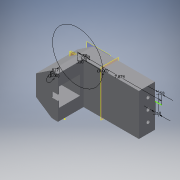
# Autodesk Inventor part: ZFrame
Saved by Autodesk Inventor 2016 (Build 200138000, 138)
## iProperties
Created: 2016-03-26
Part Number: ZFrame
Material: Generic
Document SubType Name: Modeling
Designer: Scott
Density: 1 g/cm^3
Appearance: Default
Author: Scott
Autodesk Inventor part; units mm, degrees
ref_plane "YZ Plane" through (0, 0, 0) normal (1, 0, 0) x (0, 1, 0)
ref_plane "XZ Plane" through (0, 0, 0) normal (0, 1, 0) x (-1, 0, 0)
ref_plane "XY Plane" through (0, 0, 0) normal (0, 0, 1) x (1, 0, 0)
ref_plane "Work Plane1" through (-25.4, 50.8, 0) normal (0, 1, 0) x (0, 0, -1)
ref_plane "Work Plane2" through (0, 0, 0) normal (0, 0, 1) x (1, 0, 0)
sketch "Sketch1" plane through (0, 0, 0) normal (0, 0, 1) x (1, 0, 0)
  point P0 (0, 0)
ref_plane "Work Plane3" through (0, 0, 3.175) normal (0, 0, 1) x (1, 0, 0)
sketch "Sketch2" plane through (0, 0, 3.175) normal (0, 0, 1) x (1, 0, 0)
  arc A0 (-27.2599, 1.8599) -> (-22.7697, 0) centre (-22.7697, 6.35) ccw projected
  line L0 (-27.2599, 1.8599) -> (-48.9401, 23.5401) projected
  arc A1 (-50.8, 28.0303) -> (-48.9401, 23.5401) centre (-44.45, 28.0303) ccw projected
  line L1 (-50.8, 28.0303) -> (-50.8, 48.1697) projected
  arc A2 (-48.9401, 52.6599) -> (-50.8, 48.1697) centre (-44.45, 48.1697) ccw projected
  line L2 (-48.9401, 52.6599) -> (-27.2599, 74.3401) projected
  arc A3 (-22.7697, 76.2) -> (-27.2599, 74.3401) centre (-22.7697, 69.85) ccw projected
  line L3 (-22.7697, 76.2) -> (0, 76.2) projected
  line L4 (0, 76.2) -> (0, 0) projected
  line L5 (0, 0) -> (-22.7697, 0) projected
  arc A4 (-25.4, 0.5704) -> (-22.7697, 0) centre (-22.7697, 6.35) ccw projected
  line L6 (0, 0) -> (-22.7697, 0) projected
  line L7 (0, 76.2) -> (0, 0) projected
  line L8 (0, 76.2) -> (-22.7697, 76.2) projected
  arc A5 (-22.7697, 76.2) -> (-25.4, 75.6296) centre (-22.7697, 69.85) ccw projected
  line L9 (-25.4, 57.15) -> (-25.4, 75.6296) projected
  arc A6 (-31.75, 50.8) -> (-25.4, 57.15) centre (-31.75, 57.15) ccw projected
  line L10 (-31.75, 50.8) -> (-50.2296, 50.8) projected
  arc A7 (-50.2296, 50.8) -> (-50.8, 48.1697) centre (-44.45, 48.1697) ccw projected
  line L11 (-50.8, 28.0303) -> (-50.8, 48.1697) projected
  arc A8 (-50.8, 28.0303) -> (-50.2296, 25.4) centre (-44.45, 28.0303) ccw projected
  line L12 (-31.75, 25.4) -> (-50.2296, 25.4) projected
  arc A9 (-25.4, 19.05) -> (-31.75, 25.4) centre (-31.75, 19.05) ccw projected
  line L13 (-25.4, 0.5704) -> (-25.4, 19.05) projected
  arc A10 (-22.7697, 78.74) -> (-27.94, 77.0819) centre (-22.7697, 69.85) ccw
  line L14 (-27.94, 77.0819) -> (-27.94, 57.15)
  arc A11 (-31.75, 53.34) -> (-27.94, 57.15) centre (-31.75, 57.15) ccw
  line L15 (-31.75, 53.34) -> (-51.6819, 53.34)
  line L16 (-51.6819, 22.86) -> (-31.75, 22.86)
  arc A12 (-27.94, 19.05) -> (-31.75, 22.86) centre (-31.75, 19.05) ccw
  line L17 (-27.94, 19.05) -> (-27.94, -0.8819)
  arc A13 (-27.94, -0.8819) -> (-22.7697, -2.54) centre (-22.7697, 6.35) ccw
  line L18 (-51.6819, 22.86) -> (-55.3326, 22.86)
  line L19 (-57.15, 38.1) -> (-57.15, 22.86)
  line L20 (-57.15, 22.86) -> (-55.3326, 22.86)
  line L21 (-57.15, 38.1) -> (-57.15, 53.34)
  line L22 (-57.15, 53.34) -> (-51.6819, 53.34)
  line L23 (-22.7697, -2.54) -> (0, -2.54)
  line L24 (0, -2.54) -> (117.094, -2.54)
  line L25 (-22.7697, 78.74) -> (0, 78.74)
  line L26 (0, 78.74) -> (117.094, 78.74)
  line L27 (117.094, 78.74) -> (117.094, -2.54)
  line L28 (-66.04, 62.23) -> (-66.04, 38.1)
  line L29 (-66.04, 38.1) -> (-66.04, 13.97)
  arc A14 (-36.83, -4.5329) -> (-22.7697, -11.43) centre (-22.7697, 6.35) ccw
  line L30 (-22.7697, -11.43) -> (0, -11.43)
  line L31 (0, -11.43) -> (125.984, -11.43)
  line L32 (125.984, -11.43) -> (125.984, 87.63)
  line L33 (125.984, 87.63) -> (0, 87.63)
  line L34 (0, 87.63) -> (-22.7697, 87.63)
  line L35 (-66.04, 13.97) -> (-30.6001, -9.6129)
  line L36 (-66.04, 62.23) -> (-32.6758, 84.6148)
  arc A15 (-22.7697, 87.63) -> (-32.6758, 84.6148) centre (-22.7697, 69.85) ccw
  line L37 (-48.26, 22.86) -> (-31.75, 22.86)
  line L38 (-31.75, 22.86) -> (-27.94, 19.05)
  line L39 (-27.94, 19.05) -> (-27.94, -0.8819)
  line L40 (-27.94, -0.8819) -> (-22.7697, -2.54)
  line L41 (-22.7697, 78.74) -> (-27.94, 77.0819)
  line L42 (-27.94, 77.0819) -> (-27.94, 57.15)
  line L43 (-27.94, 57.15) -> (-31.75, 53.34)
  line L44 (-31.75, 53.34) -> (-51.6819, 53.34)
  dimension "d0" = 2.54
  dimension "d1" = 2.54
  dimension "d10" = 117.094
  dimension "d11" = 180
  dimension "d12" = 117.094
  dimension "d13" = 8.89
  constraints: 62 end point, 14 point on circle, 6 centre point, 5 collinear, 4 perpendicular, 4 point on line, 2 horizontal, 2 parallel, 2 tangent, 12 other
  measures "d0" radial gap between concentric circles of A6 A11
  measures "d1" distance between parallel lines of L12 L16
  measures "d10" distance of L23.end L24.end
  measures "d11" angle of L24 L23
  measures "d12" distance of L25.end L26.end
  measures "d13" distance between parallel lines of L21 L28
ref_plane "Work Plane4" through (-20.32, 38.1, -38.1) normal (0, 0, -1) x (-1, 0, 0)
sketch "Sketch3" plane through (-20.32, 38.1, -38.1) normal (0, 0, -1) x (-1, 0, 0)
  line L0 (33.1588, 0) -> (36.9688, 0)
  line L1 (36.9688, 0) -> (45.8588, 0)
  line L2 (45.8588, 0) -> (54.7488, 0)
  line L3 (54.7488, 0) -> (-145.2512, 0)
  line L4 (-145.2512, 0) -> (-138.9012, 0)
  line L5 (-138.9012, 0) -> (-130.0112, 0)
  point P0 (-20.32, -38.1)
  dimension "d2" = 3.81
  dimension "d3" = 8.89
  dimension "d4" = 8.89
  dimension "d5" = 200
  dimension "d6" = 0
  dimension "d8" = 6.35
  dimension "d9" = 8.89
  constraints: 12 end point, 3 point on line, 2 horizontal, 1 collinear
  measures "d2" distance of L0.start L0.end
  measures "d3" distance of L0.end L1.end
  measures "d4" distance of L1.end L2.end
  measures "d5" distance of L2.end L3.end
  measures "d6" distance between parallel lines of L3 L2
  measures "d8" distance of L3.end L4.end
  measures "d9" distance of L4.end L5.end
extrude "Extrusion1" add sketch "Sketch2" against normal blind 31.75 contours L0 L17 A12 L16 A1 L12 A9 L13 A0 | L0 L16 L38 L17 | L38 A12 | L9 A6 L10 A2 L2 L15 A11 L14 A3 | L14 L43 L15 L2 | A11 L43 | L36 A15 L34 L33 L32 L31 L30 A14 L35 L29 L28
sketch "Sketch4" plane through (0, 0, -28.575) normal (0, 0, -1) x (-1, 0, 0)
  line L0 (31.75, 22.86) -> (27.94, 19.05) projected
  arc A0 (31.75, 22.86) -> (27.94, 19.05) centre (31.75, 19.05) ccw projected
  line L1 (66.04, 13.97) -> (66.04, 62.23) projected
  line L2 (66.04, 62.23) -> (32.6758, 84.6148) projected
  arc A1 (32.6758, 84.6148) -> (22.7697, 87.63) centre (22.7697, 69.85) ccw projected
  line L3 (22.7697, 87.63) -> (-125.984, 87.63) projected
  line L4 (-125.984, 87.63) -> (-125.984, -11.43) projected
  line L5 (-125.984, -11.43) -> (22.7697, -11.43) projected
  arc A2 (22.7697, -11.43) -> (30.6001, -9.6129) centre (22.7697, 6.35) ccw projected
  line L6 (30.6001, -9.6129) -> (66.04, 13.97) projected
  line L7 (27.2599, 74.3401) -> (27.94, 73.66) projected
  arc A3 (27.2599, 74.3401) -> (25.4, 75.6296) centre (22.7697, 69.85) ccw projected
  line L8 (25.4, 57.15) -> (25.4, 75.6296) projected
  arc A4 (25.4, 57.15) -> (31.75, 50.8) centre (31.75, 57.15) ccw projected
  line L9 (50.2296, 50.8) -> (31.75, 50.8) projected
  arc A5 (50.2296, 50.8) -> (48.9401, 52.6599) centre (44.45, 48.1697) ccw projected
  line L10 (48.26, 53.34) -> (48.9401, 52.6599) projected
  line L11 (48.26, 53.34) -> (57.15, 53.34) projected
  line L12 (57.15, 53.34) -> (57.15, 22.86) projected
  line L13 (57.15, 22.86) -> (48.26, 22.86) projected
  line L14 (48.9401, 23.5401) -> (48.26, 22.86) projected
  arc A6 (48.9401, 23.5401) -> (50.2296, 25.4) centre (44.45, 28.0303) ccw projected
  line L15 (31.75, 25.4) -> (50.2296, 25.4) projected
  arc A7 (31.75, 25.4) -> (25.4, 19.05) centre (31.75, 19.05) ccw projected
  line L16 (25.4, 0.5704) -> (25.4, 19.05) projected
  arc A8 (25.4, 0.5704) -> (27.2599, 1.8599) centre (22.7697, 6.35) ccw projected
  line L17 (27.94, 2.54) -> (27.2599, 1.8599) projected
  line L18 (27.94, 2.54) -> (27.94, -0.8819) projected
  arc A9 (22.7697, -2.54) -> (27.94, -0.8819) centre (22.7697, 6.35) ccw projected
  line L19 (22.7697, -2.54) -> (-117.094, -2.54) projected
  line L20 (-117.094, -2.54) -> (-117.094, 78.74) projected
  line L21 (-117.094, 78.74) -> (22.7697, 78.74) projected
  arc A10 (27.94, 77.0819) -> (22.7697, 78.74) centre (22.7697, 69.85) ccw projected
  line L22 (27.94, 77.0819) -> (27.94, 73.66) projected
  line L23 (27.94, 57.15) -> (31.75, 53.34) projected
  arc A11 (27.94, 57.15) -> (31.75, 53.34) centre (31.75, 57.15) ccw projected
  line L24 (27.94, 19.05) -> (27.94, 2.54)
  line L25 (31.75, 22.86) -> (48.26, 22.86)
  line L26 (48.26, 53.34) -> (31.75, 53.34)
  line L27 (27.94, 73.66) -> (27.94, 77.0819) projected
  line L28 (27.94, 57.15) -> (27.94, 73.66)
  point P0 (0, 0)
  constraints: 8 end point, 1 collinear, 1 horizontal, 1 perpendicular, 1 vertical
extrude "Extrusion2" cut sketch "Sketch4" against normal blind 31.75 contours A0 L24 L17 A8 L16 A7 L15 A6 L14 L25 | L10 A5 L9 A4 L8 A3 L7 L28 A11 L26
sketch "Sketch5" plane through (0, 0, -28.575) normal (0, 0, -1) x (-1, 0, 0)
  line L0 (66.04, 13.97) -> (66.04, 62.23) projected
  line L1 (66.04, 62.23) -> (32.6758, 84.6148) projected
  arc A0 (32.6758, 84.6148) -> (22.7697, 87.63) centre (22.7697, 69.85) ccw projected
  line L2 (22.7697, 87.63) -> (-125.984, 87.63) projected
  line L3 (-125.984, 87.63) -> (-125.984, -11.43) projected
  line L4 (-125.984, -11.43) -> (22.7697, -11.43) projected
  arc A1 (22.7697, -11.43) -> (30.6001, -9.6129) centre (22.7697, 6.35) ccw projected
  line L5 (30.6001, -9.6129) -> (66.04, 13.97) projected
  line L6 (57.15, 22.86) -> (31.75, 22.86) projected
  line L7 (31.75, 22.86) -> (27.94, 19.05) projected
  line L8 (27.94, 19.05) -> (27.94, -0.8819) projected
  arc A2 (22.7697, -2.54) -> (27.94, -0.8819) centre (22.7697, 6.35) ccw projected
  line L9 (22.7697, -2.54) -> (-117.094, -2.54) projected
  line L10 (-117.094, -2.54) -> (-117.094, 78.74) projected
  line L11 (-117.094, 78.74) -> (22.7697, 78.74) projected
  arc A3 (27.94, 77.0819) -> (22.7697, 78.74) centre (22.7697, 69.85) ccw projected
  line L12 (27.94, 77.0819) -> (27.94, 57.15) projected
  line L13 (27.94, 57.15) -> (31.75, 53.34) projected
  line L14 (31.75, 53.34) -> (57.15, 53.34) projected
  line L15 (57.15, 53.34) -> (57.15, 22.86) projected
  arc A4 (27.94, 57.15) -> (31.75, 53.34) centre (31.75, 57.15) ccw
  line L16 (31.75, 22.86) -> (27.94, 19.05) projected
  arc A5 (31.75, 22.86) -> (27.94, 19.05) centre (31.75, 19.05) ccw
  point P0 (0, 0)
  dimension "d18" = 3.81
  constraints: 4 point on circle, 2 centre point, 2 tangent
  measures "d18" radius of A5
extrude "Extrusion3" add sketch "Sketch5" against normal blind 31.75 contours L7 A5 | A4 L13
fillet "Fillet1" radius 3.7084 6 edges at (-29.0559, 21.7441, -28.575) (-27.94, 9.084, -28.575) (-44.45, 22.86, -28.575) (-29.0559, 54.4559, -28.575) (-27.94, 67.116, -28.575) (-40.005, 53.34, -28.575)
sketch "Sketch6" plane through (-27.94, 57.15, 3.175) normal (1, 0, 0) x (0, 0, -1)
  circle A0 centre (15.875, -44.45) radius 8 projected
  circle A1 centre (15.875, 6.35) radius 8 projected
  circle A2 centre (15.875, -44.45) radius 4
  circle A3 centre (15.875, 6.35) radius 4
  point P0 (3.175, -57.15)
  dimension "d22" = 8
  dimension "d23" = 8
  constraints: 2 centre point, 2 coincident
  measures "d22" diameter of A2
  measures "d23" diameter of A3
extrude "Extrusion4" cut sketch "Sketch6" along normal mid plane 4318 contours A2 | A3
sketch "Sketch7" plane through (117.094, -2.54, 3.175) normal (-1, 0, 0) x (0, 0, 1)
  circle A0 centre (-15.875, 40.64) radius 5.08 projected
  circle A1 centre (-15.875, 40.64) radius 4
  point P0 (-3.175, 2.54)
  dimension "d26" = 8
  constraints: 1 centre point, 1 coincident
  measures "d26" diameter of A1
extrude "Extrusion5" cut sketch "Sketch7" along normal mid plane 4318 contours A1
sketch "Sketch8" plane through (117.094, -2.54, 3.175) normal (-1, 0, 0) x (0, 0, 1)
  circle A0 centre (-15.875, 40.64) radius 4 projected
  circle A1 centre (-15.875, 15.24) radius 4 projected
  circle A2 centre (-15.875, 66.04) radius 4 projected
  line L0 (0, 81.28) -> (0, 0) projected
  line L1 (0, 81.28) -> (-31.75, 81.28) projected
  line L2 (-31.75, 0) -> (-31.75, 81.28) projected
  line L3 (0, 0) -> (-31.75, 0) projected
  circle A3 centre (-15.875, 40.64) radius 4 projected
  circle A4 centre (-15.875, 40.64) radius 6.5038
  circle A5 centre (-15.875, 40.64) radius 11
  point P0 (-3.175, 2.54)
  dimension "d29" = 22
  constraints: 2 centre point, 2 coincident
  measures "d29" diameter of A5
extrude "Extrusion6" cut sketch "Sketch8" against normal blind 7.5 contours A0 | A4 | A5
sketch "Sketch9" plane through (117.094, -2.54, 3.175) normal (-1, 0, 0) x (0, 0, 1)
  circle A0 centre (-15.875, 40.64) radius 11 projected
  circle A1 centre (-15.875, 15.24) radius 4 projected
  circle A2 centre (-15.875, 66.04) radius 4 projected
  line L0 (0, 81.28) -> (0, 0) projected
  line L1 (0, 81.28) -> (-31.75, 81.28) projected
  line L2 (-31.75, 0) -> (-31.75, 81.28) projected
  line L3 (0, 0) -> (-31.75, 0) projected
  point P0 (-3.175, 2.54)
extrude "Extrusion7" add sketch "Sketch9" along normal blind 8.89
sketch "Sketch10" plane through (125.984, -11.43, 3.175) normal (1, 0, 0) x (0, 0, -1)
  circle A0 centre (15.875, 49.53) radius 4 projected
  circle A1 centre (15.875, 24.13) radius 4 projected
  circle A2 centre (15.875, 74.93) radius 4 projected
  line L0 (0, 0) -> (0, 99.06) projected
  line L1 (0, 0) -> (31.75, 0) projected
  line L2 (31.75, 99.06) -> (31.75, 0) projected
  line L3 (0, 99.06) -> (31.75, 99.06) projected
  point P0 (3.175, 11.43)
extrude "Extrusion8" cut sketch "Sketch10" against normal blind 7.62
sketch "Sketch11" plane through (118.364, -11.43, 3.175) normal (1, 0, 0) x (0, 0, -1)
  line L0 (0, 34.29) -> (28.0416, 34.29) projected
  circle A0 centre (15.875, 49.53) radius 11 projected
  circle A1 centre (15.875, 74.93) radius 4 projected
  circle A2 centre (15.875, 24.13) radius 4 projected
  line L1 (0, 0) -> (0, 99.06) projected
  line L2 (31.75, 0) -> (0, 0) projected
  line L3 (31.75, 99.06) -> (31.75, 0) projected
  line L4 (0, 99.06) -> (31.75, 99.06) projected
  circle A3 centre (15.875, 49.53) radius 4 projected
  circle A4 centre (15.875, 49.53) radius 4
  point P0 (3.175, 11.43)
  dimension "d36" = 8
  constraints: 1 centre point, 1 coincident
  measures "d36" diameter of A4
extrude "Extrusion9" add sketch "Sketch11" against normal blind 1.39 contours A0
sketch "Sketch12" plane through (0, 0, 3.175) normal (0, 0, 1) x (1, 0, 0)
  line L0 (118.364, -11.43) -> (118.364, 87.63) projected
  line L1 (118.364, 87.63) -> (-22.7697, 87.63) projected
  arc A0 (-22.7697, 87.63) -> (-32.6758, 84.6148) centre (-22.7697, 69.85) ccw projected
  line L2 (-32.6758, 84.6148) -> (-66.04, 62.23) projected
  line L3 (-66.04, 62.23) -> (-66.04, 13.97) projected
  line L4 (-66.04, 13.97) -> (-30.6001, -9.6129) projected
  arc A1 (-30.6001, -9.6129) -> (-22.7697, -11.43) centre (-22.7697, 6.35) ccw projected
  line L5 (-22.7697, -11.43) -> (118.364, -11.43) projected
  line L6 (-31.75, 22.86) -> (-57.15, 22.86) projected
  line L7 (-57.15, 22.86) -> (-57.15, 53.34) projected
  line L8 (-57.15, 53.34) -> (-31.75, 53.34) projected
  arc A2 (-31.75, 53.34) -> (-27.94, 57.15) centre (-31.75, 57.15) ccw projected
  line L9 (-27.94, 57.15) -> (-27.94, 77.0819) projected
  arc A3 (-22.7697, 78.74) -> (-27.94, 77.0819) centre (-22.7697, 69.85) ccw projected
  line L10 (-22.7697, 78.74) -> (108.204, 78.74) projected
  line L11 (108.204, -2.54) -> (108.204, 78.74) projected
  line L12 (108.204, -2.54) -> (-22.7697, -2.54) projected
  arc A4 (-27.94, -0.8819) -> (-22.7697, -2.54) centre (-22.7697, 6.35) ccw projected
  line L13 (-27.94, -0.8819) -> (-27.94, 19.05) projected
  arc A5 (-27.94, 19.05) -> (-31.75, 22.86) centre (-31.75, 19.05) ccw projected
  point P0 (0, 0)
extrude "Extrusion10" add sketch "Sketch12" along normal blind 6.35 contours L5 A1 L4 L3 L2 A0 L1 L0 | L6 L7 L8 A2 L9 A3 L10 L11 L12 A4 L13 A5
sketch "Sketch13" plane through (-66.04, 13.97, -28.575) normal (-1, 0, 0) x (0, 0, 1)
  circle A0 centre (15.875, 24.13) radius 4 projected
  circle A1 centre (15.875, 24.13) radius 4 projected
  line L0 (15.875, 24.13) -> (72.39, 24.13)
  line L1 (96.52, 48.26) -> (48.26, 48.26)
  line L2 (48.26, 48.26) -> (48.26, 0)
  line L3 (48.26, 0) -> (96.52, 0)
  line L4 (96.52, 0) -> (96.52, 48.26)
  line L5 (96.52, 48.26) -> (48.26, 0) construction
  line L6 (48.26, 48.26) -> (96.52, 0) construction
  line L7 (72.39, 24.13) -> (89.89, 24.13)
  line L8 (89.89, 24.13) -> (54.89, 24.13)
  line L9 (54.89, 24.13) -> (89.89, 24.13) construction
  line L10 (67.39, 11.63) -> (77.39, 11.63)
  line L11 (77.39, 36.63) -> (67.39, 36.63)
  arc A2 (67.39, 36.63) -> (67.39, 11.63) centre (67.39, 24.13) ccw
  arc A3 (77.39, 11.63) -> (77.39, 36.63) centre (77.39, 24.13) ccw
  line L12 (72.39, 24.13) -> (72.39, 8.63)
  line L13 (72.39, 8.63) -> (87.89, 8.63)
  line L14 (87.89, 8.63) -> (92.89, 8.63)
  line L15 (92.89, 8.63) -> (82.89, 8.63)
  line L16 (92.89, 8.63) -> (82.89, 8.63) construction
  line L17 (91.39, 10.13) -> (84.39, 10.13)
  line L18 (84.39, 7.13) -> (91.39, 7.13)
  arc A4 (91.39, 7.13) -> (91.39, 10.13) centre (91.39, 8.63) ccw
  arc A5 (84.39, 10.13) -> (84.39, 7.13) centre (84.39, 8.63) ccw
  line L19 (41.39, 8.63) -> (56.89, 8.63)
  line L20 (17.26, 48.26) -> (65.52, 0) construction
  arc A6 (53.39, 10.13) -> (53.39, 7.13) centre (53.39, 8.63) ccw
  line L21 (60.39, 10.13) -> (53.39, 10.13)
  line L22 (61.89, 8.63) -> (51.89, 8.63)
  line L23 (61.89, 8.63) -> (51.89, 8.63) construction
  line L24 (56.89, 8.63) -> (61.89, 8.63)
  arc A7 (60.39, 7.13) -> (60.39, 10.13) centre (60.39, 8.63) ccw
  line L25 (53.39, 7.13) -> (60.39, 7.13)
  line L26 (72.39, 39.63) -> (87.89, 39.63)
  line L27 (48.26, 79.26) -> (96.52, 31) construction
  arc A8 (84.39, 41.13) -> (84.39, 38.13) centre (84.39, 39.63) ccw
  line L28 (91.39, 41.13) -> (84.39, 41.13)
  line L29 (92.89, 39.63) -> (82.89, 39.63)
  line L30 (92.89, 39.63) -> (82.89, 39.63) construction
  line L31 (87.89, 39.63) -> (92.89, 39.63)
  arc A9 (91.39, 38.13) -> (91.39, 41.13) centre (91.39, 39.63) ccw
  line L32 (84.39, 38.13) -> (91.39, 38.13)
  line L33 (41.39, 39.63) -> (56.89, 39.63)
  line L34 (17.26, 79.26) -> (65.52, 31) construction
  arc A10 (53.39, 41.13) -> (53.39, 38.13) centre (53.39, 39.63) ccw
  line L35 (60.39, 41.13) -> (53.39, 41.13)
  line L36 (61.89, 39.63) -> (51.89, 39.63)
  line L37 (61.89, 39.63) -> (51.89, 39.63) construction
  line L38 (56.89, 39.63) -> (61.89, 39.63)
  arc A11 (60.39, 38.13) -> (60.39, 41.13) centre (60.39, 39.63) ccw
  line L39 (53.39, 38.13) -> (60.39, 38.13)
  point P0 (28.575, -13.97)
  dimension "d41" = 56.515
  dimension "d42" = 48.26
  dimension "d43" = 48.26
  dimension "d44" = 17.5
  dimension "d45" = 35
  dimension "d47" = 15.5
  dimension "d51" = 3
  dimension "d54" = 31
  dimension "d57" = 31
  constraints: 90 end point, 30 point on circle, 19 point on line, 10 centre point, 8 tangent, 5 horizontal, 4 midpoint, 4 parallel, 3 collinear, 2 perpendicular, 1 vertical, 65 other
  measures "d41" distance of L0.start L0.end
  measures "d42" distance of L3.end L2.end
  measures "d43" distance of L2.end L1.end
  measures "d44" distance of L0.end L7.end
  measures "d45" distance of L7.end L8.end
  measures "d47" distance of L12.start L12.end
  measures "d51" diameter of A5
  measures "d54" distance of L12.end L19.start
  measures "d57" distance of L12.end L26.start
extrude "Extrusion11" add sketch "Sketch13" against normal blind 2.54 contours L2 L1 L4 L3
sketch "Sketch14" plane through (-66.04, 13.97, -28.575) normal (-1, 0, 0) x (0, 0, 1)
  line L0 (96.52, 0) -> (48.26, 0) projected
  line L1 (38.1, 48.26) -> (38.1, 0) projected
  line L2 (48.26, 0) -> (38.1, 0)
  line L3 (38.1, 0) -> (38.1, 48.26)
  line L4 (38.1, 48.26) -> (48.26, 48.26)
  line L5 (48.26, 48.26) -> (48.26, 0)
  point P0 (28.575, -13.97)
  constraints: 8 end point, 3 perpendicular, 1 horizontal
extrude "Extrusion12" add sketch "Sketch14" against normal blind 2.54
sketch "Sketch15" plane through (0, 0, 9.525) normal (0, 0, 1) x (1, 0, 0)
  line L0 (-63.5, 13.97) -> (-66.04, 13.97) projected
  line L1 (-66.04, 13.97) -> (-30.6001, -9.6129) projected
  arc A0 (-30.6001, -9.6129) -> (-22.7697, -11.43) centre (-22.7697, 6.35) ccw projected
  line L2 (-22.7697, -11.43) -> (118.364, -11.43) projected
  line L3 (118.364, -11.43) -> (118.364, 87.63) projected
  line L4 (118.364, 87.63) -> (-22.7697, 87.63) projected
  arc A1 (-22.7697, 87.63) -> (-32.6758, 84.6148) centre (-22.7697, 69.85) ccw projected
  line L5 (-32.6758, 84.6148) -> (-66.04, 62.23) projected
  line L6 (-66.04, 62.23) -> (-63.5, 62.23) projected
  line L7 (-63.5, 62.23) -> (-63.5, 13.97) projected
  line L8 (-66.04, 13.97) -> (-66.04, 62.23) projected
  line L9 (-63.5, 62.23) -> (-63.5, 13.97) projected
  line L10 (-66.04, 13.97) -> (-63.5, 13.97)
  line L11 (-66.04, 16.7) -> (-27.94, 16.7) projected
  line L12 (-63.5, 13.97) -> (-13.5, 13.97)
  line L13 (-63.5, 13.97) -> (-13.5, 13.97) construction
  line L14 (-13.5, 13.97) -> (-13.5, -11.43)
  line L15 (118.364, -11.43) -> (-22.7697, -11.43) projected
  line L16 (-13.5, -11.43) -> (-13.5, 87.63)
  line L17 (-22.7697, 87.63) -> (118.364, 87.63) projected
  point P0 (0, 0)
  dimension "d64" = 50
  dimension "d65" = 0
  constraints: 10 end point, 3 point on line, 2 horizontal, 1 collinear, 1 parallel, 1 perpendicular
  measures "d64" distance of L0.start L12.end
  measures "d65" distance between parallel lines of L12 L13
sketch "Sketch16" plane through (-63.5, 13.97, -28.575) normal (1, 0, 0) x (0, 0, -1)
  arc A0 (-77.39, 36.63) -> (-77.39, 11.63) centre (-77.39, 24.13) ccw projected
  line L0 (-77.39, 36.63) -> (-67.39, 36.63) projected
  arc A1 (-67.39, 11.63) -> (-67.39, 36.63) centre (-67.39, 24.13) ccw projected
  line L1 (-67.39, 11.63) -> (-77.39, 11.63) projected
  arc A2 (-53.39, 38.13) -> (-53.39, 41.13) centre (-53.39, 39.63) ccw projected
  line L2 (-53.39, 38.13) -> (-60.39, 38.13) projected
  arc A3 (-60.39, 41.13) -> (-60.39, 38.13) centre (-60.39, 39.63) ccw projected
  line L3 (-60.39, 41.13) -> (-53.39, 41.13) projected
  arc A4 (-84.39, 38.13) -> (-84.39, 41.13) centre (-84.39, 39.63) ccw projected
  line L4 (-84.39, 38.13) -> (-91.39, 38.13) projected
  arc A5 (-91.39, 41.13) -> (-91.39, 38.13) centre (-91.39, 39.63) ccw projected
  line L5 (-91.39, 41.13) -> (-84.39, 41.13) projected
  arc A6 (-53.39, 7.13) -> (-53.39, 10.13) centre (-53.39, 8.63) ccw projected
  line L6 (-53.39, 7.13) -> (-60.39, 7.13) projected
  arc A7 (-60.39, 10.13) -> (-60.39, 7.13) centre (-60.39, 8.63) ccw projected
  line L7 (-60.39, 10.13) -> (-53.39, 10.13) projected
  arc A8 (-84.39, 7.13) -> (-84.39, 10.13) centre (-84.39, 8.63) ccw projected
  line L8 (-84.39, 7.13) -> (-91.39, 7.13) projected
  arc A9 (-91.39, 10.13) -> (-91.39, 7.13) centre (-91.39, 8.63) ccw projected
  line L9 (-91.39, 10.13) -> (-84.39, 10.13) projected
  line L10 (-38.1, 48.26) -> (-96.52, 48.26) projected
  line L11 (-96.52, 48.26) -> (-96.52, 0) projected
  line L12 (-96.52, 0) -> (-38.1, 0) projected
  line L13 (-38.1, 48.26) -> (-38.1, 0) projected
  line L14 (-67.39, 24.13) -> (-46.39, 24.13)
  line L15 (-67.39, 24.13) -> (-46.39, 24.13) construction
  point P0 (-28.575, -13.97)
  dimension "d66" = 21
  dimension "d67" = 0
  constraints: 4 end point, 2 horizontal, 1 collinear
  measures "d66" distance of L14.start L14.end
  measures "d67" distance between parallel lines of L14 L15
extrude "Extrusion13" add sketch "Sketch15" along normal blind 8.255
sketch "Sketch17" plane through (0, 0, 17.78) normal (0, 0, 1) x (1, 0, 0)
  line L0 (-66.04, 13.97) -> (-63.5, 13.97) projected
  line L1 (-66.04, 13.97) -> (-30.6001, -9.6129) projected
  arc A0 (-30.6001, -9.6129) -> (-22.7697, -11.43) centre (-22.7697, 6.35) ccw projected
  line L2 (-22.7697, -11.43) -> (118.364, -11.43) projected
  line L3 (118.364, -11.43) -> (118.364, 87.63) projected
  line L4 (118.364, 87.63) -> (-22.7697, 87.63) projected
  arc A1 (-22.7697, 87.63) -> (-32.6758, 84.6148) centre (-22.7697, 69.85) ccw projected
  line L5 (-32.6758, 84.6148) -> (-66.04, 62.23) projected
  line L6 (-63.5, 62.23) -> (-66.04, 62.23) projected
  line L7 (-63.5, 13.97) -> (-63.5, 62.23) projected
  line L8 (-63.5, 62.23) -> (-63.5, 13.97) projected
  line L9 (-63.5, 13.97) -> (-13.5, 13.97)
  line L10 (-27.94, 19.05) -> (-27.94, -0.8819) projected
  line L11 (-63.5, 13.97) -> (-13.5, 13.97) construction
  line L12 (118.364, -11.43) -> (-22.7697, -11.43) projected
  line L13 (-22.7697, 87.63) -> (118.364, 87.63) projected
  line L14 (-13.5, -11.43) -> (118.364, -11.43)
  line L15 (118.364, -11.43) -> (118.364, 87.63)
  line L16 (118.364, 87.63) -> (-13.5, 87.63)
  line L17 (-13.5, 87.63) -> (-13.5, -11.43)
  point P0 (0, 0)
  dimension "d70" = 50
  dimension "d71" = 0
  constraints: 12 end point, 2 horizontal, 2 parallel, 2 perpendicular, 1 collinear, 1 point on line
  measures "d70" distance of L0.end L9.end
  measures "d71" distance between parallel lines of L11 L9
extrude "Extrusion14" cut sketch "Sketch17" against normal blind 8.255 contours L17 L4 L3 L2
sketch "Sketch18" plane through (0, 0, 17.78) normal (0, 0, 1) x (1, 0, 0)
  line L0 (-13.5, -11.43) -> (-13.5, 87.63) projected
  line L1 (-13.5, 87.63) -> (-22.7697, 87.63) projected
  arc A0 (-22.7697, 87.63) -> (-32.6758, 84.6148) centre (-22.7697, 69.85) ccw projected
  line L2 (-32.6758, 84.6148) -> (-66.04, 62.23) projected
  line L3 (-63.5, 62.23) -> (-66.04, 62.23) projected
  line L4 (-63.5, 13.97) -> (-63.5, 62.23) projected
  line L5 (-66.04, 13.97) -> (-63.5, 13.97) projected
  line L6 (-66.04, 13.97) -> (-30.6001, -9.6129) projected
  arc A1 (-30.6001, -9.6129) -> (-22.7697, -11.43) centre (-22.7697, 6.35) ccw projected
  line L7 (-22.7697, -11.43) -> (-13.5, -11.43) projected
  line L8 (-63.5, 62.23) -> (-63.5, 13.97) projected
  line L9 (-11.6166, 60.6) -> (-63.5, 60.6)
  line L10 (-63.5, 60.6) -> (-63.5, 15.6)
  line L11 (-63.5, 15.6) -> (-11.6166, 15.6)
  line L12 (-11.6166, 15.6) -> (-11.6166, 60.6)
  line L13 (-11.6166, 60.6) -> (-63.5, 15.6) construction
  line L14 (-63.5, 60.6) -> (-11.6166, 15.6) construction
  point P0 (0, 0)
  point P1 (-37.5583, 38.1)
  dimension "d74" = 45
  constraints: 12 end point, 2 midpoint, 2 parallel, 1 horizontal, 1 perpendicular, 1 point on line
  measures "d74" distance of L10.end L9.end
extrude "Extrusion15" add sketch "Sketch18" along normal up to surface (50.165 mm away) contours L7 A1 L6 L5 L4 L11 L0 | L11 L4 L9 L0 | L9 L4 L3 L2 A0 L1 L0
sketch "Sketch19" plane through (-66.04, 13.97, 67.945) normal (0, 0, 1) x (1, 0, 0)
  line L0 (52.54, 73.66) -> (52.54, -25.4) projected
  line L1 (2.54, 48.26) -> (2.54, 0) projected
  line L2 (2.54, 36.63) -> (2.54, 11.63) projected
  line L3 (79.82, 46.13) -> (2.54, 46.13)
  line L4 (2.54, 46.13) -> (2.54, 2.13)
  line L5 (2.54, 2.13) -> (79.82, 2.13)
  line L6 (79.82, 2.13) -> (79.82, 46.13)
  line L7 (79.82, 46.13) -> (2.54, 2.13) construction
  line L8 (2.54, 46.13) -> (79.82, 2.13) construction
  point P0 (66.04, -13.97)
  point P1 (41.18, 24.13)
  dimension "d77" = 44
  constraints: 12 end point, 2 midpoint, 2 parallel, 1 horizontal, 1 perpendicular, 1 point on line
  measures "d77" distance of L4.end L3.end
extrude "Extrusion16" cut sketch "Sketch19" against normal blind 50.165
sketch "Sketch20" plane through (-66.04, 13.97, 67.945) normal (0, 0, 1) x (1, 0, 0)
  line L0 (40.64, 43.18) -> (40.64, 61.6596) projected
  point P0 (66.04, -13.97)
sketch "Sketch21" plane through (-66.04, 13.97, 67.945) normal (0, 0, 1) x (1, 0, 0)
  line L0 (2.54, 46.13) -> (52.54, 46.13) projected
  line L1 (52.54, 73.66) -> (52.54, 46.13) projected
  line L2 (43.2703, 73.66) -> (52.54, 73.66) projected
  arc A0 (43.2703, 73.66) -> (33.3642, 70.6448) centre (43.2703, 55.88) ccw projected
  line L3 (0, 48.26) -> (33.3642, 70.6448) projected
  line L4 (0, 0) -> (0, 48.26) projected
  line L5 (35.4399, -23.5829) -> (0, 0) projected
  arc A1 (35.4399, -23.5829) -> (43.2703, -25.4) centre (43.2703, -7.62) ccw projected
  line L6 (52.54, -25.4) -> (43.2703, -25.4) projected
  line L7 (52.54, 2.13) -> (52.54, -25.4) projected
  line L8 (52.54, 2.13) -> (2.54, 2.13) projected
  line L9 (2.54, 2.13) -> (2.54, 46.13) projected
  line L10 (52.54, 2.13) -> (2.54, 2.13) projected
  line L11 (52.54, 2.13) -> (52.54, 46.13)
  line L12 (174.244, -16.51) -> (43.2703, -16.51) projected
  point P0 (66.04, -13.97)
  constraints: 2 end point, 1 perpendicular
extrude "Extrusion17" add sketch "Sketch21" along normal blind 2.54
sketch "Sketch22" plane through (-66.04, 13.97, 70.485) normal (0, 0, 1) x (1, 0, 0)
  line L0 (52.54, -25.4) -> (52.54, 73.66) projected
  line L1 (52.54, 73.66) -> (43.2703, 73.66) projected
  arc A0 (43.2703, 73.66) -> (33.3642, 70.6448) centre (43.2703, 55.88) ccw projected
  line L2 (33.3642, 70.6448) -> (0, 48.26) projected
  line L3 (0, 48.26) -> (0, 0) projected
  line L4 (0, 0) -> (35.4399, -23.5829) projected
  arc A1 (35.4399, -23.5829) -> (43.2703, -25.4) centre (43.2703, -7.62) ccw projected
  line L5 (43.2703, -25.4) -> (52.54, -25.4) projected
  line L6 (37.54, 30.63) -> (67.54, 30.63)
  line L7 (67.54, 30.63) -> (67.54, 17.63)
  line L8 (67.54, 17.63) -> (37.54, 17.63)
  line L9 (37.54, 17.63) -> (37.54, 30.63)
  line L10 (37.54, 30.63) -> (67.54, 17.63) construction
  line L11 (67.54, 30.63) -> (37.54, 17.63) construction
  point P0 (66.04, -13.97)
  point P1 (52.54, 24.13)
  dimension "d82" = 30
  dimension "d83" = 13
  constraints: 12 end point, 3 midpoint, 2 parallel, 1 horizontal, 1 perpendicular
  measures "d82" distance of L7.end L8.end
  measures "d83" distance of L6.end L7.end
extrude "Extrusion18" cut sketch "Sketch22" against normal blind 7.3025 contours L8 L9 L6 L0 | L0 L6 L7 L8
ref_plane "Work Plane5" through (29.464, -11.43, 3.175) normal (1, 0, 0) x (0, 0, -1)
sketch "Sketch23" plane through (-57.15, 19.1516, -28.575) normal (1, 0, 0) x (0, 0, -1)
  circle A0 centre (-15.875, 18.9484) radius 4 projected
  circle A1 centre (-15.875, 18.9484) radius 11
  point P0 (-28.575, -19.1516)
  dimension "d87" = 22
  constraints: 1 centre point, 1 coincident
  measures "d87" diameter of A1
extrude "Extrusion19" cut sketch "Sketch23" against normal blind 7.5 contours A0 | A1
ref_plane "Work Plane6" through (29.464, -11.43, 3.175) normal (1, 0, 0) x (0, 0, -1)
body "Solid1"
